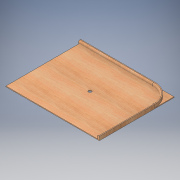
# Autodesk Inventor part: ShooterBase
Saved by Autodesk Inventor 2016 (Build 200138000, 138)
## iProperties
Created: 2015-07-21
Part Number: ShooterBase
Material: Wood (Birch)
Document SubType Name: Modeling
Designer: steele
Density: 0.55 g/cm^3
Appearance: Birch - Natural Polished
Mass: 2597.87 g
Surface Area: 10546.3 cm^2
Volume: 4723.41 cm^3
Author: steele
Autodesk Inventor part; units mm, degrees
ref_plane "YZ Plane" through (0, 0, 0) normal (1, 0, 0) x (0, 1, 0)
ref_plane "XZ Plane" through (0, 0, 0) normal (0, 1, 0) x (-1, 0, 0)
ref_plane "XY Plane" through (0, 0, 0) normal (0, 0, 1) x (1, 0, 0)
sketch "Sketch1" plane through (0, 0, 0) normal (0, 1, 0) x (-1, 0, 0)
  line L0 (-381, 304.8) -> (-381, -304.8)
  line L1 (-381, -304.8) -> (381, -304.8)
  line L2 (381, -304.8) -> (381, 304.8)
  line L3 (381, 304.8) -> (-381, 304.8)
  line L4 (-381, 304.8) -> (381, -304.8) construction
  line L5 (-381, -304.8) -> (381, 304.8) construction
  point P0 (0, 0)
  dimension "width" = 609.6
  dimension "length" = 762
  constraints: 12 end point, 2 midpoint, 2 parallel, 1 perpendicular, 1 vertical
  measures "width" distance of L0.start L0.end
  measures "length" distance of L2.end L0.start
extrude "Extrusion1" add sketch "Sketch1" against normal blind 6.35
ref_plane "Work Plane3" through (-381, 0, 304.8) normal (0, 0, 1) x (1, 0, 0)
sketch "Sketch5" plane through (-381, 0, 304.8) normal (0, 0, 1) x (1, 0, 0)
  line L0 (762, 0) -> (755.65, 0)
  line L1 (755.65, 25.4) -> (762, 25.4)
  line L2 (762, 25.4) -> (762, 0)
  arc A0 (755.65, 25.4) -> (755.65, 0) centre (755.65, 12.7) ccw
  point P0 (381, 0)
  dimension "d16" = 25.4
  constraints: 6 end point, 2 point on circle, 1 centre point, 1 horizontal, 1 parallel
  measures "d16" distance of L1.end L0.start
ref_plane "Work Plane4" through (0, 12.7, 0) normal (0, 1, 0) x (1, 0, 0)
sketch "Sketch6" plane through (0, 12.7, 0) normal (0, 1, 0) x (1, 0, 0)
  line L0 (-381, 304.8) -> (381, 304.8) construction
  line L1 (222.25, 304.8) -> (222.25, 146.05) construction
  line L2 (222.25, 146.05) -> (381, 146.05) construction
  line L3 (381, 304.8) -> (381, -304.8) construction
  arc A0 (368.3, 146.05) -> (222.25, 292.1) centre (222.25, 146.05) ccw
  line L4 (222.25, 292.1) -> (-381, 292.1)
  line L5 (-381, -304.8) -> (-381, 304.8) projected
  line L6 (368.3, 146.05) -> (368.3, -304.8)
  line L7 (381, -304.8) -> (-381, -304.8) projected
  point P0 (0, 0)
  dimension "d20" = 158.75
  dimension "diameterOfFrisbee" = 292.1
  constraints: 8 end point, 6 point on line, 2 perpendicular, 2 point on circle, 2 vertical, 1 centre point, 1 coincident, 1 horizontal
  measures "d20" distance of L1.start L1.end
  measures "diameterOfFrisbee" diameter of A0
sweep "Sweep2" add profiles "Sketch5" path "Sketch6" path curves L6 A0 L4
sketch "Sketch7" plane through (0, 0, 0) normal (0, 1, 0) x (1, 0, 0)
  point P0 (0, 0)
  point P1 (0, 0)
  constraints: 1 coincident
hole "Hole1" at (0, 0, 0) direction (0, -1, 0) diameter 25.4 end through all
body "Solid1"
